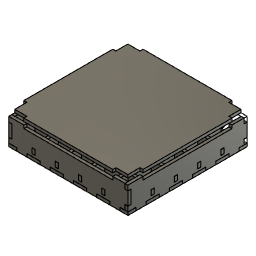
artisan box laser v1 (Autodesk Fusion 360 design; units mm, degrees)
Autodesk Fusion 360 part; units mm, degrees
note: some values were not read from the file. Set by a fixed rule: which sketch regions a step uses.
sketch "bottom" plane through (0, 0, 0) normal (0, 1, 0) x (1, 0, 0)
  line L0 (117.05, 70.05) -> (113.95, 70.05)
  line L1 (117.05, 59.95) -> (113.95, 59.95)
  line L2 (94.05, 59.95) -> (90.95, 59.95)
  line L3 (94.05, 70.05) -> (90.95, 70.05)
  line L4 (71.05, 59.95) -> (67.95, 59.95)
  line L5 (71.05, 70.05) -> (67.95, 70.05)
  line L6 (48.05, 59.95) -> (44.95, 59.95)
  line L7 (48.05, 70.05) -> (44.95, 70.05)
  line L8 (117.05, 36.95) -> (113.95, 36.95)
  line L9 (117.05, 47.05) -> (113.95, 47.05)
  line L10 (94.05, 47.05) -> (90.95, 47.05)
  line L11 (94.05, 36.95) -> (90.95, 36.95)
  line L12 (71.05, 36.95) -> (67.95, 36.95)
  line L13 (71.05, 47.05) -> (67.95, 47.05)
  line L14 (48.05, 47.05) -> (44.95, 47.05)
  line L15 (48.05, 36.95) -> (44.95, 36.95)
  line L16 (117.05, 24.05) -> (113.95, 24.05)
  line L17 (117.05, 13.95) -> (113.95, 13.95)
  line L18 (94.05, 13.95) -> (90.95, 13.95)
  line L19 (94.05, 24.05) -> (90.95, 24.05)
  line L20 (71.05, 24.05) -> (67.95, 24.05)
  line L21 (71.05, 13.95) -> (67.95, 13.95)
  line L22 (48.05, 13.95) -> (44.95, 13.95)
  line L23 (48.05, 24.05) -> (44.95, 24.05)
  line L24 (117.05, 1.05) -> (113.95, 1.05)
  line L25 (117.05, -9.05) -> (113.95, -9.05)
  line L26 (94.05, -9.05) -> (90.95, -9.05)
  line L27 (94.05, 1.05) -> (90.95, 1.05)
  line L28 (71.05, 1.05) -> (67.95, 1.05)
  line L29 (71.05, -9.05) -> (67.95, -9.05)
  line L30 (48.05, -9.05) -> (44.95, -9.05)
  line L31 (48.05, 1.05) -> (44.95, 1.05)
  line L32 (117.05, -21.95) -> (113.95, -21.95)
  line L33 (117.05, -32.05) -> (113.95, -32.05)
  line L34 (94.05, -32.05) -> (90.95, -32.05)
  line L35 (94.05, -21.95) -> (90.95, -21.95)
  line L36 (71.05, -21.95) -> (67.95, -21.95)
  line L37 (71.05, -32.05) -> (67.95, -32.05)
  line L38 (48.05, -32.05) -> (44.95, -32.05)
  line L39 (48.05, -21.95) -> (44.95, -21.95)
  line L40 (132, 55.05) -> (132, 52)
  line L41 (122, 55.05) -> (122, 52)
  line L42 (109.05, 55) -> (109.05, 52)
  line L43 (98.95, 55.05) -> (98.95, 52)
  line L44 (86, 55.05) -> (86, 51.95)
  line L45 (76, 55) -> (76, 52)
  line L46 (63.05, 55) -> (63.05, 52)
  line L47 (53, 55) -> (53, 52)
  line L48 (40.05, 55) -> (40.05, 52)
  line L49 (29.95, 55) -> (29.95, 51.95)
  line L50 (75.95, 32.05) -> (75.95, 28.95)
  line L51 (29.95, 32.05) -> (29.95, 28.95)
  line L52 (63.05, 32.05) -> (63.05, 28.95)
  line L53 (52.95, 32.05) -> (52.95, 28.95)
  line L54 (40.05, 32.05) -> (40.05, 28.95)
  line L55 (132.05, 32.05) -> (132.05, 28.95)
  line L56 (98.95, 32.05) -> (98.95, 28.95)
  line L57 (86.05, 32.05) -> (86.05, 28.95)
  line L58 (121.95, 32.05) -> (121.95, 28.95)
  line L59 (109.05, 32.05) -> (109.05, 28.95)
  line L60 (75.95, 55.05) -> (75.95, 51.95)
  line L61 (30, 55.05) -> (30, 52)
  line L62 (63, 55.05) -> (63, 51.95)
  line L63 (52.95, 55.05) -> (52.95, 51.95)
  line L64 (40, 55.05) -> (40, 51.95)
  line L65 (132.05, 55) -> (132.05, 51.95)
  line L66 (99, 55) -> (99, 51.95)
  line L67 (86.05, 55) -> (86.05, 52)
  line L68 (121.95, 55) -> (121.95, 51.95)
  line L69 (109, 55.05) -> (109, 51.95)
  line L70 (75.95, 9.05) -> (75.95, 5.95)
  line L71 (29.95, 9.05) -> (29.95, 5.95)
  line L72 (63.05, 9.05) -> (63.05, 5.95)
  line L73 (52.95, 9.05) -> (52.95, 5.95)
  line L74 (40.05, 9.05) -> (40.05, 5.95)
  line L75 (132.05, 9.05) -> (132.05, 5.95)
  line L76 (98.95, 9.05) -> (98.95, 5.95)
  line L77 (86.05, 9.05) -> (86.05, 5.95)
  line L78 (121.95, 9.05) -> (121.95, 5.95)
  line L79 (109.05, 9.05) -> (109.05, 5.95)
  line L80 (75.95, -13.95) -> (75.95, -17)
  line L81 (29.95, -13.95) -> (29.95, -17.05)
  line L82 (63.05, -13.95) -> (63.05, -17.05)
  line L83 (52.95, -13.95) -> (52.95, -17.05)
  line L84 (40.05, -13.95) -> (40.05, -17.05)
  line L85 (132.05, -13.95) -> (132.05, -17.05)
  line L86 (98.95, -13.95) -> (98.95, -17.05)
  line L87 (86.05, -13.95) -> (86.05, -17.05)
  line L88 (121.95, -13.95) -> (121.95, -17.05)
  line L89 (109.05, -13.95) -> (109.05, -17.05)
  line L90 (29.95, 78) -> (29.95, 75)
  line L91 (75.95, 78) -> (75.95, 75)
  line L92 (40.05, 78) -> (40.05, 75)
  line L93 (52.95, 78) -> (52.95, 75)
  line L94 (132.05, 78) -> (132.05, 75)
  line L95 (121.95, 78) -> (121.95, 75)
  line L96 (63.05, 78) -> (63.05, 75)
  line L97 (109.05, 78) -> (109.05, 75)
  line L98 (86.05, 78) -> (86.05, 75)
  line L99 (98.95, 78) -> (98.95, 75)
  line L100 (63.05, -37) -> (63.05, -40)
  line L101 (52.95, -37) -> (52.95, -40)
  line L102 (40.05, -37) -> (40.05, -40)
  line L103 (75.95, -37) -> (75.95, -40)
  line L104 (86.05, -37) -> (86.05, -40)
  line L105 (29.95, -37) -> (29.95, -40)
  line L106 (132.05, -37) -> (132.05, -40)
  line L107 (121.95, -37) -> (121.95, -40)
  line L108 (109.05, -37) -> (109.05, -40)
  line L109 (98.95, -37) -> (98.95, -40)
  line L110 (140, 47.05) -> (137, 47.05)
  line L111 (140, 13.95) -> (137, 13.95)
  line L112 (140, 24.05) -> (137, 24.05)
  line L113 (140, 1.05) -> (137, 1.05)
  line L114 (140, -32.05) -> (137, -32.05)
  line L115 (140, -21.95) -> (137, -21.95)
  line L116 (140, -9.05) -> (137, -9.05)
  line L117 (140, 36.95) -> (137, 36.95)
  line L118 (140, 59.95) -> (137, 59.95)
  line L119 (140, 70.05) -> (137, 70.05)
  line L120 (25, 47.05) -> (22, 47.05)
  line L121 (25, 13.95) -> (22, 13.95)
  line L122 (25, 24.05) -> (22, 24.05)
  line L123 (25, 1.05) -> (22, 1.05)
  line L124 (25, -32.05) -> (22, -32.05)
  line L125 (25, -21.95) -> (22, -21.95)
  line L126 (25, -9.05) -> (22, -9.05)
  line L127 (25, 36.95) -> (22, 36.95)
  line L128 (25, 59.95) -> (22, 59.95)
  line L129 (25, 70.05) -> (22, 70.05)
  line L130 (22, 70.05) -> (22, 78)
  line L131 (22, 78) -> (29.95, 78)
  line L132 (40, 78) -> (52.95, 78)
  line L133 (63, 78) -> (75.95, 78)
  line L134 (86, 78) -> (98.95, 78)
  line L135 (109.05, 78) -> (121.95, 78)
  line L136 (132, 78) -> (140, 78)
  line L137 (140, 78) -> (140, 70.05)
  line L138 (140, 59.95) -> (140, 47.05)
  line L139 (140, 36.95) -> (140, 24.05)
  line L140 (140, 13.95) -> (140, 1.05)
  line L141 (140, -9.05) -> (140, -21.95)
  line L142 (140, -32.05) -> (140, -40)
  line L143 (140, -40) -> (132, -40)
  line L144 (122, -40) -> (109, -40)
  line L145 (98.95, -40) -> (86, -40)
  line L146 (75.95, -40) -> (63.05, -40)
  line L147 (53, -40) -> (40, -40)
  line L148 (29.95, -40) -> (22, -40)
  line L149 (22, -40) -> (22, -32.05)
  line L150 (22, -21.95) -> (22, -9.05)
  line L151 (22, 1.05) -> (22, 13.95)
  line L152 (22, 24.05) -> (22, 36.95)
  line L153 (22, 47.05) -> (22, 59.95)
  line L154 (113.95, 70.05) -> (113.95, 59.95)
  line L155 (98.95, 55.05) -> (109, 55.05)
  line L156 (94.05, 70.05) -> (94.05, 59.95)
  line L157 (90.95, 70.05) -> (90.95, 59.95)
  line L158 (86, 55.05) -> (75.95, 55.05)
  line L159 (71.05, 70.05) -> (71.05, 59.95)
  line L160 (29.95, 75) -> (40.05, 75)
  line L161 (52.95, 75) -> (63.05, 75)
  line L162 (67.95, 70.05) -> (67.95, 59.95)
  line L163 (48.05, 70.05) -> (48.05, 59.95)
  line L164 (44.95, 70.05) -> (44.95, 59.95)
  line L165 (25, 70.05) -> (25, 59.95)
  line L166 (30, 55.05) -> (40, 55.05)
  line L167 (52.95, 55.05) -> (63, 55.05)
  line L168 (122, 55.05) -> (132, 55.05)
  line L169 (137, 59.95) -> (137, 70.05)
  line L170 (117.05, 70.05) -> (117.05, 59.95)
  line L171 (25, 47.05) -> (25, 36.95)
  line L172 (29.95, 32.05) -> (40.05, 32.05)
  line L173 (40, 51.95) -> (29.95, 51.95)
  line L174 (52.95, 51.95) -> (63, 51.95)
  line L175 (75.95, 51.95) -> (86, 51.95)
  line L176 (99, 51.95) -> (109, 51.95)
  line L177 (121.95, 51.95) -> (132.05, 51.95)
  line L178 (137, 47.05) -> (137, 36.95)
  line L179 (132.05, 32.05) -> (121.95, 32.05)
  line L180 (117.05, 36.95) -> (117.05, 47.05)
  line L181 (113.95, 47.05) -> (113.95, 36.95)
  line L182 (109.05, 32.05) -> (98.95, 32.05)
  line L183 (94.05, 36.95) -> (94.05, 47.05)
  line L184 (90.95, 47.05) -> (90.95, 36.95)
  line L185 (86.05, 32.05) -> (75.95, 32.05)
  line L186 (71.05, 36.95) -> (71.05, 47.05)
  line L187 (67.95, 47.05) -> (67.95, 36.95)
  line L188 (63.05, 32.05) -> (52.95, 32.05)
  line L189 (48.05, 36.95) -> (48.05, 47.05)
  line L190 (44.95, 47.05) -> (44.95, 36.95)
  line L191 (137, 24.05) -> (137, 13.95)
  line L192 (132.05, 28.95) -> (121.95, 28.95)
  line L193 (132.05, 9.05) -> (121.95, 9.05)
  line L194 (117.05, 13.95) -> (117.05, 24.05)
  line L195 (113.95, 24.05) -> (113.95, 13.95)
  line L196 (109.05, 9.05) -> (98.95, 9.05)
  line L197 (98.95, 28.95) -> (109.05, 28.95)
  line L198 (94.05, 24.05) -> (94.05, 13.95)
  line L199 (90.95, 13.95) -> (90.95, 24.05)
  line L200 (86.05, 28.95) -> (75.95, 28.95)
  line L201 (86.05, 9.05) -> (75.95, 9.05)
  line L202 (71.05, 13.95) -> (71.05, 24.05)
  line L203 (67.95, 24.05) -> (67.95, 13.95)
  line L204 (63.05, 9.05) -> (52.95, 9.05)
  line L205 (52.95, 28.95) -> (63.05, 28.95)
  line L206 (48.05, 24.05) -> (48.05, 13.95)
  line L207 (44.95, 13.95) -> (44.95, 24.05)
  line L208 (40.05, 28.95) -> (29.95, 28.95)
  line L209 (40.05, 9.05) -> (29.95, 9.05)
  line L210 (25, 13.95) -> (25, 24.05)
  line L211 (137, -9.05) -> (137, 1.05)
  line L212 (132.05, 5.95) -> (121.95, 5.95)
  line L213 (132.05, -13.95) -> (121.95, -13.95)
  line L214 (117.05, -9.05) -> (117.05, 1.05)
  line L215 (113.95, 1.05) -> (113.95, -9.05)
  line L216 (109.05, -13.95) -> (98.95, -13.95)
  line L217 (98.95, 5.95) -> (109.05, 5.95)
  line L218 (94.05, 1.05) -> (94.05, -9.05)
  line L219 (90.95, -9.05) -> (90.95, 1.05)
  line L220 (86.05, 5.95) -> (75.95, 5.95)
  line L221 (86.05, -13.95) -> (75.95, -13.95)
  line L222 (71.05, -9.05) -> (71.05, 1.05)
  line L223 (67.95, 1.05) -> (67.95, -9.05)
  line L224 (63.05, -13.95) -> (52.95, -13.95)
  line L225 (52.95, 5.95) -> (63.05, 5.95)
  line L226 (48.05, 1.05) -> (48.05, -9.05)
  line L227 (44.95, 1.05) -> (44.95, -9.05)
  line L228 (40.05, -13.95) -> (29.95, -13.95)
  line L229 (29.95, 5.95) -> (40.05, 5.95)
  line L230 (25, 1.05) -> (25, -9.05)
  line L231 (25, -21.95) -> (25, -32.05)
  line L232 (29.95, -17.05) -> (40.05, -17.05)
  line L233 (29.95, -37) -> (40.05, -37)
  line L234 (44.95, -21.95) -> (44.95, -32.05)
  line L235 (48.05, -21.95) -> (48.05, -32.05)
  line L236 (52.95, -17.05) -> (63.05, -17.05)
  line L237 (52.95, -37) -> (63.05, -37)
  line L238 (67.95, -32.05) -> (67.95, -21.95)
  line L239 (71.05, -21.95) -> (71.05, -32.05)
  line L240 (76, -17.05) -> (86.05, -17.05)
  line L241 (90.95, -21.95) -> (90.95, -32.05)
  line L242 (94.05, -21.95) -> (94.05, -32.05)
  line L243 (98.95, -17.05) -> (109.05, -17.05)
  line L244 (113.95, -32.05) -> (113.95, -21.95)
  line L245 (117.05, -21.95) -> (117.05, -32.05)
  line L246 (121.95, -17.05) -> (132.05, -17.05)
  line L247 (137, -32.05) -> (137, -21.95)
  line L248 (86.05, 75) -> (75.95, 75)
  line L249 (75.95, -37) -> (86.05, -37)
  line L250 (98.95, -37) -> (109.05, -37)
  line L251 (121.95, -37) -> (132.05, -37)
  line L252 (109.05, 75) -> (98.95, 75)
  line L253 (121.95, 75) -> (132.05, 75)
  constraint perpendicular L129 L130
  constraint perpendicular L91 L133
  constraint perpendicular L99 L134
  constraint perpendicular L95 L135
  constraint perpendicular L94 L136
  constraint perpendicular L119 L137
  constraint perpendicular L110 L138
  constraint perpendicular L112 L139
  constraint perpendicular L113 L140
  constraint perpendicular L115 L141
  constraint perpendicular L114 L142
  constraint perpendicular L109 L145
  constraint perpendicular L101 L147
  constraint perpendicular L105 L148
  constraint perpendicular L126 L150
  constraint perpendicular L121 L151
  constraint perpendicular L122 L152
  constraint perpendicular L120 L153
  constraint perpendicular L1 L154
  constraint perpendicular L69 L155
  constraint perpendicular L2 L156
  constraint perpendicular L2 L157
  constraint perpendicular L45 L158
  constraint perpendicular L4 L159
  constraint perpendicular L90 L160
  constraint perpendicular L4 L162
  constraint perpendicular L7 L163
  constraint perpendicular L6 L164
  constraint perpendicular L128 L165
  constraint perpendicular L61 L166
  constraint perpendicular L46 L167
  constraint perpendicular L65 L168
  constraint perpendicular L119 L169
  constraint perpendicular L1 L170
  constraint perpendicular L127 L171
  constraint perpendicular L54 L172
  constraint perpendicular L49 L173
  constraint perpendicular L46 L174
  constraint perpendicular L60 L175
  constraint perpendicular L69 L176
  constraint perpendicular L40 L177
  constraint perpendicular L117 L178
  constraint perpendicular L58 L179
  constraint perpendicular L8 L180
  constraint perpendicular L8 L181
  constraint perpendicular L56 L182
  constraint perpendicular L10 L183
  constraint perpendicular L11 L184
  constraint perpendicular L50 L185
  constraint perpendicular L13 L186
  constraint perpendicular L12 L187
  constraint perpendicular L52 L188
  constraint perpendicular L14 L189
  constraint perpendicular L15 L190
  constraint perpendicular L111 L191
  constraint perpendicular L55 L192
  constraint perpendicular L78 L193
  constraint perpendicular L16 L194
  constraint perpendicular L17 L195
  constraint perpendicular L76 L196
  constraint perpendicular L59 L197
  constraint perpendicular L18 L198
  constraint perpendicular L19 L199
  constraint perpendicular L57 L200
  constraint perpendicular L77 L201
  constraint perpendicular L20 L202
  constraint perpendicular L20 L203
  constraint perpendicular L73 L204
  constraint perpendicular L52 L205
  constraint perpendicular L22 L206
  constraint perpendicular L23 L207
  constraint perpendicular L51 L208
  constraint perpendicular L71 L209
  constraint perpendicular L121 L210
  constraint perpendicular L116 L211
  constraint perpendicular L78 L212
  constraint perpendicular L88 L213
  constraint perpendicular L24 L214
  constraint perpendicular L25 L215
  constraint perpendicular L86 L216
  constraint perpendicular L79 L217
  constraint perpendicular L27 L218
  constraint perpendicular L27 L219
  constraint perpendicular L70 L220
  constraint perpendicular L80 L221
  constraint perpendicular L28 L222
  constraint perpendicular L29 L223
  constraint perpendicular L83 L224
  constraint perpendicular L73 L225
  constraint perpendicular L30 L226
  constraint perpendicular L30 L227
  constraint perpendicular L84 L228
  constraint perpendicular L74 L229
  constraint perpendicular L126 L230
  constraint perpendicular L124 L231
  constraint perpendicular L84 L232
  constraint perpendicular L39 L234
  constraint perpendicular L39 L235
  constraint perpendicular L83 L236
  constraint perpendicular L36 L238
  constraint perpendicular L37 L239
  constraint perpendicular L34 L241
  constraint perpendicular L34 L242
  constraint perpendicular L89 L243
  constraint perpendicular L32 L244
  constraint perpendicular L33 L245
  constraint perpendicular L85 L246
  constraint perpendicular L115 L247
  constraint perpendicular L91 L248
  constraint perpendicular L103 L249
  constraint perpendicular L108 L250
  constraint perpendicular L106 L251
  constraint perpendicular L99 L252
  constraint perpendicular L94 L253
extrude "Extrude1" add sketch "bottom" along normal blind 3 makes body 1
sketch "dividers" plane through (0, 0, 0) normal (0, 1, 0) x (1, 0, 0)
  line L0 (150, 75) -> (150, 70)
  line L1 (150, 70) -> (147, 70)
  line L2 (147, 70) -> (147, 60)
  line L3 (147, 60) -> (150, 60)
  line L4 (150, 47) -> (147, 47)
  line L5 (147, 47) -> (147, 37)
  line L6 (147, 37) -> (150, 37)
  line L7 (150, 24) -> (147, 24)
  line L8 (147, 24) -> (147, 14)
  line L9 (147, 14) -> (150, 14)
  line L10 (150, 1) -> (147, 1)
  line L11 (147, 1) -> (147, -9)
  line L12 (147, -9) -> (150, -9)
  line L13 (150, -22) -> (147, -22)
  line L14 (147, -22) -> (147, -32)
  line L15 (147, -32) -> (150, -32)
  line L16 (150, -32) -> (150, -37)
  line L17 (160, -37) -> (160, 75)
  line L18 (150, 60) -> (150, 55)
  line L19 (150, 55) -> (155, 55)
  line L20 (155, 55) -> (155, 52)
  line L21 (155, 52) -> (150, 52)
  line L22 (150, 52) -> (150, 47)
  line L23 (150, 37) -> (150, 32)
  line L24 (150, 32) -> (155, 32)
  line L25 (155, 32) -> (155, 29)
  line L26 (155, 29) -> (150, 29)
  line L27 (150, 29) -> (150, 24)
  line L28 (150, 14) -> (150, 9)
  line L29 (150, 9) -> (155, 9)
  line L30 (155, 9) -> (155, 6)
  line L31 (155, 6) -> (150, 6)
  line L32 (150, 6) -> (150, 1)
  line L33 (150, -9) -> (150, -14)
  line L34 (150, -14) -> (155, -14)
  line L35 (155, -14) -> (155, -17)
  line L36 (155, -17) -> (150, -17)
  line L37 (150, -17) -> (150, -22)
  line L38 (167, 37) -> (170, 37)
  line L39 (167, -32) -> (170, -32)
  line L40 (170, 1) -> (167, 1)
  line L41 (167, 1) -> (167, -9)
  line L42 (170, 24) -> (167, 24)
  line L43 (175, 9) -> (175, 6)
  line L44 (167, 24) -> (167, 14)
  line L45 (175, 55) -> (175, 52)
  line L46 (175, 32) -> (175, 29)
  line L47 (167, 14) -> (170, 14)
  line L48 (170, -32) -> (170, -37)
  line L49 (167, 47) -> (167, 37)
  line L50 (167, 70) -> (167, 60)
  line L51 (170, 75) -> (170, 70)
  line L52 (175, -14) -> (175, -17)
  line L53 (170, 70) -> (167, 70)
  line L54 (167, 60) -> (170, 60)
  line L55 (170, -22) -> (167, -22)
  line L56 (167, -22) -> (167, -32)
  line L57 (167, -9) -> (170, -9)
  line L58 (170, 47) -> (167, 47)
  line L59 (175, 55) -> (180, 55)
  line L60 (175, 52) -> (180, 52)
  line L61 (175, 32) -> (180, 32)
  line L62 (175, 29) -> (180, 29)
  line L63 (175, 9) -> (180, 9)
  line L64 (175, 6) -> (180, 6)
  line L65 (175, -14) -> (180, -14)
  line L66 (175, -17) -> (180, -17)
  line L67 (170, 60) -> (170, 47)
  line L68 (170, 37) -> (170, 24)
  line L69 (170, 14) -> (170, 1)
  line L70 (170, -9) -> (170, -22)
  line L71 (180, -37) -> (180, -17)
  line L72 (180, -14) -> (180, 6)
  line L73 (180, 9) -> (180, 29)
  line L74 (180, 32) -> (180, 52)
  line L75 (180, 55) -> (180, 75)
  line L76 (150, 75) -> (152.5, 75)
  line L77 (152.5, 75) -> (152.5, 78)
  line L78 (152.5, 78) -> (157.5, 78)
  line L79 (157.5, 78) -> (157.5, 75)
  line L80 (157.5, 75) -> (160, 75)
  line L81 (170, 75) -> (172.5, 75)
  line L82 (172.5, 75) -> (172.5, 78)
  line L83 (172.5, 78) -> (177.5, 78)
  line L84 (177.5, 78) -> (177.5, 75)
  line L85 (177.5, 75) -> (180, 75)
  line L86 (150, -37) -> (152.5, -37)
  line L87 (152.5, -37) -> (152.5, -40)
  line L88 (152.5, -40) -> (157.5, -40)
  line L89 (157.5, -40) -> (157.5, -37)
  line L90 (157.5, -37) -> (160, -37)
  line L91 (170, -37) -> (172.5, -37)
  line L92 (172.5, -37) -> (172.5, -40)
  line L93 (172.5, -40) -> (177.5, -40)
  line L94 (177.5, -40) -> (177.5, -37)
  line L95 (177.5, -37) -> (180, -37)
  constraint vertical L0
  constraint perpendicular L0 L1
  constraint perpendicular L1 L2
  constraint perpendicular L2 L3
  constraint perpendicular L4 L5
  constraint perpendicular L5 L6
  constraint perpendicular L6 L8
  constraint perpendicular L10 L11
  constraint perpendicular L11 L12
  constraint perpendicular L11 L13
  constraint perpendicular L13 L14
  constraint perpendicular L14 L15
  constraint perpendicular L15 L16
  constraint perpendicular L3 L18
  constraint perpendicular L18 L19
  constraint perpendicular L19 L20
  constraint perpendicular L18 L21
  constraint perpendicular L4 L22
  constraint perpendicular L6 L23
  constraint perpendicular L23 L24
  constraint perpendicular L6 L25
  constraint perpendicular L25 L26
  constraint perpendicular L7 L27
  constraint perpendicular L9 L28
  constraint perpendicular L28 L29
  constraint perpendicular L29 L30
  constraint perpendicular L30 L31
  constraint perpendicular L10 L32
  constraint perpendicular L12 L33
  constraint perpendicular L33 L34
  constraint perpendicular L34 L35
  constraint perpendicular L35 L36
  constraint perpendicular L13 L37
  constraint vertical L51
  constraint perpendicular L51 L53
  constraint perpendicular L50 L53
  constraint perpendicular L50 L54
  constraint perpendicular L49 L58
  constraint perpendicular L38 L49
  constraint perpendicular L38 L44
  constraint perpendicular L40 L41
  constraint perpendicular L41 L57
  constraint perpendicular L41 L55
  constraint perpendicular L55 L56
  constraint perpendicular L39 L56
  constraint perpendicular L39 L48
  constraint perpendicular L38 L46
  constraint perpendicular L45 L60
  constraint perpendicular L43 L63
  constraint perpendicular L54 L67
  constraint perpendicular L42 L68
  constraint perpendicular L40 L69
  constraint perpendicular L55 L70
  constraint perpendicular L66 L71
  constraint perpendicular L62 L73
  constraint perpendicular L61 L74
  constraint perpendicular L17 L76
  constraint perpendicular L76 L77
  constraint perpendicular L77 L78
  constraint perpendicular L78 L79
  constraint perpendicular L17 L80
  constraint perpendicular L51 L81
  constraint perpendicular L81 L82
  constraint perpendicular L82 L83
  constraint perpendicular L81 L84
  constraint parallel L83 L85
  constraint perpendicular L16 L86
  constraint perpendicular L86 L87
  constraint perpendicular L87 L88
  constraint perpendicular L88 L89
  constraint perpendicular L17 L90
  constraint perpendicular L48 L91
  constraint perpendicular L91 L92
  constraint perpendicular L92 L93
  constraint perpendicular L93 L94
  constraint perpendicular L71 L95
extrude "Extrude2" add sketch "dividers" along normal blind 3 separate body makes body 2 at (176.6667, 0, -20.6667) makes body 3 at (155, 0, 25.3333)
move_body "Move1" bodies 3 to x (0, 1, 0) y (-1, 0, 0) z (0, 0, 1) at (147, -147, 0)
move_body "Move2" bodies 2 to x (0, 1, 0) y (-1, 0, 0) z (0, 0, 1) at (167, -167, 0)
move_body "Move3" bodies 2 to x (1, 0, 0) y (0, 1, 0) z (0, 0, 1) at (-50, 0, -0.05)
copy_body "CopyPasteBodies1" bodies 2 makes body 4
move_body "Move4" bodies 4 to x (1, 0, 0) y (0, 1, 0) z (0, 0, 1) at (-23, 0, 0)
copy_body "CopyPasteBodies2" bodies 2 makes body 5
move_body "Move5" bodies 5 to x (1, 0, 0) y (0, 1, 0) z (0, 0, 1) at (-46, 0, 0)
copy_body "CopyPasteBodies3" bodies 2 makes body 6
move_body "Move6" bodies 6 to x (1, 0, 0) y (0, 1, 0) z (0, 0, 1) at (-69, 0, 0)
move_body "Move7" bodies 3 to x (0, 0, -1) y (0, 1, 0) z (1, 0, 0) at (222, 0, 66)
move_body "Move8" bodies 3 to x (1, 0, 0) y (0, 1, 0) z (0, 0, 1) at (-122, 0, 26)
copy_body "CopyPasteBodies4" bodies 3 makes body 7
move_body "Move9" bodies 7 to x (1, 0, 0) y (0, 1, 0) z (0, 0, 1) at (0, 0, 23)
copy_body "CopyPasteBodies5" bodies 3 makes body 8
move_body "Move10" bodies 8 to x (1, 0, 0) y (0, 1, 0) z (0, 0, 1) at (0, 0, 46)
copy_body "CopyPasteBodies6" bodies 3 makes body 9
move_body "Move11" bodies 9 to x (1, 0, 0) y (0, 1, 0) z (0, 0, 1) at (0, 0, 69)
sketch "outside walls" plane through (0, 0, 39.95) normal (0, 0, 1) x (1, 0, 0)
  line L0 (30, 0) -> (30, 3)
  line L1 (30, 0) -> (40, 0)
  line L2 (40, 0) -> (40, 3)
  line L3 (40, 3) -> (53, 3)
  line L4 (53, 3) -> (53, 0)
  line L5 (53, 0) -> (63, 0)
  line L6 (63, 0) -> (63, 3)
  line L7 (63, 3) -> (76, 3)
  line L8 (76, 3) -> (76, 0)
  line L9 (76, 0) -> (86, 0)
  line L10 (86, 0) -> (86, 3)
  line L11 (86, 3) -> (99, 3)
  line L12 (99, 3) -> (99, 0)
  line L13 (99, 0) -> (109, 0)
  line L14 (109, 0) -> (109, 3)
  line L15 (109, 3) -> (122, 3)
  line L16 (122, 3) -> (122, 0)
  line L17 (122, 0) -> (132, 0)
  line L18 (132, 0) -> (132, 3)
  line L19 (132, 3) -> (137, 3)
  line L20 (30, 3) -> (22, 3)
  line L21 (22, 26) -> (22, 21.05)
  line L22 (22, 21.05) -> (25, 21.05)
  line L23 (25, 21.05) -> (25, 7.95)
  line L24 (25, 7.95) -> (22, 7.95)
  line L25 (22, 7.95) -> (22, 3)
  line L26 (137, 3) -> (137, 8)
  line L27 (137, 8) -> (140, 8)
  line L28 (140, 8) -> (140, 21)
  line L29 (140, 21) -> (137, 21)
  line L30 (137, 21) -> (137, 26)
  line L31 (22, 26) -> (36.95, 26)
  line L32 (36.95, 26) -> (36.95, 22.9)
  line L33 (137, 26) -> (125.05, 26)
  line L34 (125.05, 26) -> (125.05, 22.9)
  line L35 (125.05, 22.9) -> (36.95, 22.9)
  line L36 (44.95, 10.55) -> (48.05, 10.55)
  line L37 (48.05, 10.55) -> (48.05, 5.45)
  line L38 (48.05, 5.45) -> (44.95, 5.45)
  line L39 (44.95, 5.45) -> (44.95, 10.55)
  line L40 (67.95, 10.55) -> (71.05, 10.55)
  line L41 (71.05, 10.55) -> (71.05, 5.45)
  line L42 (71.05, 5.45) -> (67.95, 5.45)
  line L43 (67.95, 5.45) -> (67.95, 10.55)
  line L44 (90.95, 10.55) -> (94.05, 10.55)
  line L45 (94.05, 10.55) -> (94.05, 5.45)
  line L46 (94.05, 5.45) -> (90.95, 5.45)
  line L47 (90.95, 5.45) -> (90.95, 10.55)
  line L48 (113.95, 10.55) -> (117.05, 10.55)
  line L49 (117.05, 10.55) -> (117.05, 5.45)
  line L50 (117.05, 5.45) -> (113.95, 5.45)
  line L51 (113.95, 5.45) -> (113.95, 10.55)
  constraint vertical L0
  constraint perpendicular L0 L1
  constraint perpendicular L1 L2
  constraint perpendicular L2 L3
  constraint perpendicular L3 L4
  constraint perpendicular L4 L5
  constraint perpendicular L5 L6
  constraint perpendicular L6 L7
  constraint perpendicular L7 L8
  constraint perpendicular L8 L9
  constraint perpendicular L9 L10
  constraint perpendicular L10 L11
  constraint perpendicular L11 L12
  constraint perpendicular L12 L13
  constraint perpendicular L11 L14
  constraint perpendicular L14 L15
  constraint perpendicular L11 L16
  constraint perpendicular L14 L17
  constraint perpendicular L17 L18
  constraint perpendicular L18 L19
  constraint perpendicular L0 L20
  constraint perpendicular L21 L22
  constraint perpendicular L21 L24
  constraint perpendicular L24 L25
  constraint perpendicular L19 L26
  constraint perpendicular L26 L27
  constraint perpendicular L19 L28
  constraint perpendicular L26 L29
  constraint perpendicular L21 L31
  constraint perpendicular L31 L32
  constraint perpendicular L30 L33
  constraint perpendicular L33 L34
  constraint horizontal L36
  constraint vertical L37
  constraint horizontal L38
  constraint vertical L39
  constraint horizontal L40
  constraint vertical L41
  constraint horizontal L42
  constraint vertical L43
  constraint horizontal L44
  constraint vertical L45
  constraint horizontal L46
  constraint vertical L47
  constraint horizontal L48
  constraint vertical L49
  constraint horizontal L50
  constraint vertical L51
extrude "Extrude3" add sketch "outside walls" along normal blind 3 separate body makes body 10
move_body "Move12" bodies 10 to x (1, 0, 0) y (0, 1, 0) z (0, 0, 1) at (0, 0, -3)
copy_body "CopyPasteBodies7" bodies 10 makes body 11
move_body "Move13" bodies 11 to x (0, 0, -1) y (0, 1, 0) z (1, 0, 0) at (100, 0, 62)
copy_body "CopyPasteBodies8" bodies 10 makes body 12
move_body "Move14" bodies 12 to x (-1, 0, 0) y (0, 1, 0) z (0, 0, -1) at (162, 0, -38)
copy_body "CopyPasteBodies9" bodies 10 makes body 13
move_body "Move15" bodies 13 to x (0, 0, 1) y (0, 1, 0) z (-1, 0, 0) at (62, 0, -100)
sketch "lid" plane through (0, 26, 0) normal (0, 1, 0) x (-1, 0, 0)
  line L0 (-124.95, 40.05) -> (-124.95, 37)
  line L1 (-124.95, 37) -> (-136.9, 37)
  line L2 (-139.95, -62.95) -> (-136.9, -62.95)
  line L3 (-136.9, -62.95) -> (-136.9, -74.9)
  line L4 (-136.9, -74.9) -> (-124.95, -74.9)
  line L5 (-124.95, -74.9) -> (-124.95, -77.95)
  line L6 (-124.95, -77.95) -> (-36.95, -77.95)
  line L7 (-36.95, -77.95) -> (-36.95, -74.9)
  line L8 (-36.95, -74.9) -> (-25, -74.9)
  line L9 (-25, -74.9) -> (-25, -62.95)
  line L10 (-25, -62.95) -> (-21.95, -62.95)
  line L11 (-21.95, -62.95) -> (-21.95, 25.05)
  line L12 (-21.95, 25.05) -> (-25, 25.05)
  line L13 (-25, 25.05) -> (-25, 37)
  line L14 (-25, 37) -> (-36.95, 37)
  line L15 (-36.95, 37) -> (-36.95, 40.05)
  line L16 (-36.95, 40.05) -> (-124.95, 40.05)
  line L17 (-136.9, 37) -> (-136.9, 25.05)
  line L18 (-136.9, 25.05) -> (-139.95, 25.05)
  line L19 (-139.95, 25.05) -> (-139.95, -62.95)
  constraint perpendicular L0 L1
  constraint perpendicular L2 L3
  constraint perpendicular L3 L4
  constraint perpendicular L4 L5
  constraint perpendicular L5 L6
  constraint perpendicular L4 L7
  constraint perpendicular L7 L8
  constraint perpendicular L4 L9
  constraint perpendicular L9 L10
  constraint perpendicular L10 L11
  constraint perpendicular L11 L12
  constraint perpendicular L12 L13
  constraint perpendicular L13 L14
  constraint perpendicular L14 L15
  constraint perpendicular L0 L16
  constraint perpendicular L1 L17
  constraint perpendicular L17 L18
  constraint perpendicular L2 L19
extrude "Extrude4" add sketch "lid" against normal blind 3 separate body makes body 14
move_body "Move16" bodies 14 to x (1, 0, 0) y (0, 1, 0) z (0, 0, 1) at (0, 6, 0)
move_body "Move17" bodies 3 to x (1, 0, 0) y (0, 1, 0) z (0, 0, 1) at (0.1, 0, 0)
named bodies: "bottom", "divider top", "divider bottom", "divider top (1)", "divider top (1) (1)", "divider top (2)", "divider bottom (1)", "divider bottom (1) (1)", "divider bottom (2)", "outside walls", "outside walls (1)", "outside walls (1) (1)", "outside walls (2)", "lid"
